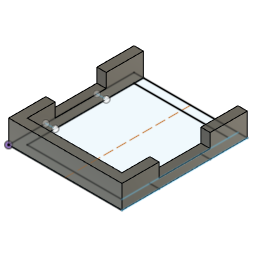
Final Project (Autodesk Fusion 360 design; units mm, degrees)
Autodesk Fusion 360 part; units mm, degrees
sketch "Sketch1" plane through (0, 0, 0) normal (0, 0, 1) x (1, 0, 0)
  line L0 (0, 0) -> (70, 0)
  line L1 (70, 0) -> (70, 120)
  line L2 (70, 120) -> (0, 120)
  line L3 (0, 120) -> (0, 0)
  dimension "d1" = 70
  dimension "d2" = 120
  constraint horizontal L0
  constraint vertical L1
  constraint horizontal L2
  constraint vertical L3
  constraint coincident L0.start L3.end
  measures "d1" distance of L0.start L0.end
  measures "d2" distance of L0.start L2.end
extrude "Extrude1" add sketch "Sketch1" along normal blind 25 makes body 1
sketch "Sketch2" plane through (0, 0, 25) normal (0, 0, 1) x (-1, 0, 0)
  line L0 (0, -120) -> (0, 0)
  line L1 (0, 0) -> (-70, 0)
  line L2 (-70, 0) -> (-70, -120)
  line L3 (-70, -120) -> (0, -120)
  line L4 (-5, -115) -> (-65, -115)
  line L5 (-65, -115) -> (-65, -5)
  line L6 (-65, -5) -> (-5, -5)
  line L7 (-5, -5) -> (-5, -115)
  dimension "d5" = 60
  dimension "d6" = 110
  dimension "d7" = 5
  dimension "d8" = 5
  constraint horizontal L4
  constraint vertical L5
  constraint horizontal L6
  constraint vertical L7
  measures "d5" distance of L4.start L4.end
  measures "d6" distance of L4.start L6.end
  measures "d7" distance of L2 L5
  measures "d8" distance of L1 L6
extrude "Extrude2" cut sketch "Sketch2" against normal blind 5 contours L4 L5 L6 L7 bodies 1
shell "Shell1" thickness 3 removed faces 1 at (23.3333, 80, 0) on bodies 1
sketch "Plate Sketch" plane through (0, 0, 17) normal (0, 0, -1) x (1, 0, 0)
  line L0 (3, -3) -> (3, -117)
  line L1 (3, -117) -> (67, -117)
  line L2 (67, -117) -> (67, -3)
  line L3 (67, -3) -> (3, -3)
  line L4 (8.9, -24) -> (23.1, -24)
  line L5 (23.1, -24) -> (23.1, -9.8)
  line L6 (23.1, -9.8) -> (8.9, -9.8)
  line L7 (8.9, -9.8) -> (8.9, -24)
  line L8 (3, -81) -> (67, -81) construction
  line L9 (61.1, -117) -> (61.1, -3) construction
  line L10 (27.9, -9.8) -> (27.9, -24)
  line L11 (27.9, -24) -> (42.1, -24)
  line L12 (42.1, -24) -> (42.1, -9.8)
  line L13 (42.1, -9.8) -> (27.9, -9.8)
  line L14 (46.9, -9.8) -> (46.9, -24)
  line L15 (46.9, -24) -> (61.1, -24)
  line L16 (61.1, -24) -> (61.1, -9.8)
  line L17 (61.1, -9.8) -> (46.9, -9.8)
  line L18 (8.9, -28.8) -> (8.9, -43)
  line L19 (8.9, -43) -> (23.1, -43)
  line L20 (23.1, -43) -> (23.1, -28.8)
  line L21 (23.1, -28.8) -> (8.9, -28.8)
  line L22 (27.9, -28.8) -> (27.9, -43)
  line L23 (27.9, -43) -> (42.1, -43)
  line L24 (42.1, -43) -> (42.1, -28.8)
  line L25 (42.1, -28.8) -> (27.9, -28.8)
  line L26 (46.9, -28.8) -> (46.9, -43)
  line L27 (46.9, -43) -> (61.1, -43)
  line L28 (61.1, -43) -> (61.1, -28.8)
  line L29 (61.1, -28.8) -> (46.9, -28.8)
  line L30 (8.9, -47.8) -> (8.9, -62)
  line L31 (8.9, -62) -> (23.1, -62)
  line L32 (23.1, -62) -> (23.1, -47.8)
  line L33 (23.1, -47.8) -> (8.9, -47.8)
  line L34 (27.9, -47.8) -> (27.9, -62)
  line L35 (27.9, -62) -> (42.1, -62)
  line L36 (42.1, -62) -> (42.1, -47.8)
  line L37 (42.1, -47.8) -> (27.9, -47.8)
  line L38 (46.9, -47.8) -> (46.9, -62)
  line L39 (46.9, -62) -> (61.1, -62)
  line L40 (61.1, -62) -> (61.1, -47.8)
  line L41 (61.1, -47.8) -> (46.9, -47.8)
  line L42 (8.9, -66.8) -> (8.9, -81)
  line L43 (8.9, -81) -> (23.1, -81)
  line L44 (23.1, -81) -> (23.1, -66.8)
  line L45 (23.1, -66.8) -> (8.9, -66.8)
  line L46 (27.9, -66.8) -> (27.9, -81)
  line L47 (27.9, -81) -> (42.1, -81)
  line L48 (42.1, -81) -> (42.1, -66.8)
  line L49 (42.1, -66.8) -> (27.9, -66.8)
  line L50 (46.9, -66.8) -> (46.9, -81)
  line L51 (46.9, -81) -> (61.1, -81)
  line L52 (61.1, -81) -> (61.1, -66.8)
  line L53 (61.1, -66.8) -> (46.9, -66.8)
  line L54 (46.9, -106.3141) -> (61.1, -106.3141)
  line L55 (61.1, -106.3141) -> (61.1, -92.1141)
  line L56 (61.1, -92.1141) -> (46.9, -92.1141)
  line L57 (46.9, -92.1141) -> (46.9, -106.3141)
  line L58 (46.9, -106.3141) -> (61.1, -92.1141) construction
  line L59 (61.1, -106.3141) -> (46.9, -92.1141) construction
  circle A0 centre (54, -99.2141) radius 3.5
  line L60 (9.0541, -114.2194) -> (34.0541, -114.2194) construction
  line L61 (34.0541, -114.2194) -> (34.0541, -87.2194) construction
  line L62 (34.0541, -87.2194) -> (9.0541, -87.2194) construction
  line L63 (9.0541, -87.2194) -> (9.0541, -114.2194) construction
  dimension "d18" = 14.2
  dimension "d19" = 14.2
  dimension "d20" = 6.8
  dimension "d21" = 5.9
  dimension "d23" = 5.9
  dimension "d24" = 71.2
  dimension "d27" = 38
  dimension "d28" = -57
  dimension "d29" = 14.2
  dimension "d30" = 14.2
  dimension "d32" = 5.9
  dimension "d33" = 7
  dimension "d34" = 25
  dimension "d35" = 27
  constraint horizontal L4
  constraint vertical L5
  constraint horizontal L6
  constraint vertical L7
  constraint coincident L0 L8.start
  constraint coincident L2 L8.end
  constraint perpendicular L2 L8
  constraint coincident L1 L9.start
  constraint coincident L3 L9.end
  constraint perpendicular L3 L9
  constraint horizontal L54
  constraint vertical L55
  constraint horizontal L56
  constraint vertical L57
  constraint midpoint L59 A0.centre
  constraint horizontal L60
  constraint vertical L61
  constraint horizontal L62
  constraint vertical L63
  measures "d18" distance of L4.start L4.end
  measures "d19" distance of L4.start L6.end
  measures "d20" distance of L3 L6
  measures "d21" distance of L0 L7
  measures "d23" distance of L2 L9
  measures "d24" distance of L6 L8
  measures "d29" distance of L54.start L54.end
  measures "d30" distance of L54.start L56.end
  measures "d32" distance of L2 L55
  measures "d33" diameter of A0
  measures "d34" distance of L60.start L60.end
  measures "d35" distance of L60.start L62.end
extrude "Extrude3" cut sketch "Plate Sketch" against normal blind 3 contours L0 L1 L2 L3 | L4 L5 L6 L7 | L10 L11 L12 L13 | L14 L15 L16 L17 | L18 L19 L20 L21 | L22 L23 L24 L25 | L26 L27 L28 L29 | L30 L31 L32 L33 | L34 L35 L36 L37 | L38 L39 L40 L41 | L42 L43 L44 L45 | L46 L47 L48 L49 | L50 L51 L52 L53 | L54 L55 L56 L57 | A0 bodies 1
extrude "Extrude4" add sketch "Plate Sketch" against normal blind 3 separate body contours L0 L1 L2 L3 | L54 L55 L56 L57 makes body 2
extrude "Extrude9" add 1 faces at (23.3333, 0, 8.3333) along direction (0, -1, 0) blind 5 on bodies 1 bodies 1
extrude "Extrude10" add 1 faces at (46.6667, 120, 8.3333) along direction (0, 1, 0) blind 5 on bodies 1 bodies 1
extrude "Extrude11" add 1 faces at (24.3333, 122.3333, 0) along direction (0, 0, -1) blind 2 separate body on bodies 1 makes body 3
extrude "Extrude12" add 1 faces at (24.3333, 117, -0.6667) along direction (0, -1, 0) blind 114 on bodies 3 bodies 3
sketch "Base Sketch" plane through (0, 0, 0) normal (0, 0, 1) x (-1, 0, 0)
  line L0 (0, -125) -> (0, 5)
  line L1 (0, 5) -> (-70, 5)
  line L2 (-70, 5) -> (-70, -125)
  line L3 (-70, -125) -> (0, -125)
  line L4 (-61.1, -66.8) -> (-46.9, -66.8)
  line L5 (-46.9, -66.8) -> (-46.9, -81)
  line L6 (-46.9, -81) -> (-61.1, -81)
  line L7 (-61.1, -81) -> (-61.1, -66.8)
  circle A0 centre (-54, -99.2141) radius 3.5
  line L8 (-23.1, -66.8) -> (-8.9, -66.8)
  line L9 (-8.9, -66.8) -> (-8.9, -81)
  line L10 (-8.9, -81) -> (-23.1, -81)
  line L11 (-23.1, -81) -> (-23.1, -66.8)
  line L12 (-23.1, -47.8) -> (-8.9, -47.8)
  line L13 (-8.9, -47.8) -> (-8.9, -62)
  line L14 (-8.9, -62) -> (-23.1, -62)
  line L15 (-23.1, -62) -> (-23.1, -47.8)
  line L16 (-42.1, -28.8) -> (-27.9, -28.8)
  line L17 (-27.9, -28.8) -> (-27.9, -43)
  line L18 (-27.9, -43) -> (-42.1, -43)
  line L19 (-42.1, -43) -> (-42.1, -28.8)
  line L20 (-42.1, -9.8) -> (-27.9, -9.8)
  line L21 (-27.9, -9.8) -> (-27.9, -24)
  line L22 (-27.9, -24) -> (-42.1, -24)
  line L23 (-42.1, -24) -> (-42.1, -9.8)
  line L24 (-23.1, -28.8) -> (-8.9, -28.8)
  line L25 (-8.9, -28.8) -> (-8.9, -43)
  line L26 (-8.9, -43) -> (-23.1, -43)
  line L27 (-23.1, -43) -> (-23.1, -28.8)
  line L28 (-61.1, -9.8) -> (-46.9, -9.8)
  line L29 (-46.9, -9.8) -> (-46.9, -24)
  line L30 (-46.9, -24) -> (-61.1, -24)
  line L31 (-61.1, -24) -> (-61.1, -9.8)
  line L32 (-8.9, -9.8) -> (-8.9, -24)
  line L33 (-8.9, -24) -> (-23.1, -24)
  line L34 (-23.1, -24) -> (-23.1, -9.8)
  line L35 (-23.1, -9.8) -> (-8.9, -9.8)
  line L36 (-61.1, -28.8) -> (-46.9, -28.8)
  line L37 (-46.9, -28.8) -> (-46.9, -43)
  line L38 (-46.9, -43) -> (-61.1, -43)
  line L39 (-61.1, -43) -> (-61.1, -28.8)
  line L40 (-61.1, -47.8) -> (-46.9, -47.8)
  line L41 (-46.9, -47.8) -> (-46.9, -62)
  line L42 (-46.9, -62) -> (-61.1, -62)
  line L43 (-61.1, -62) -> (-61.1, -47.8)
  line L44 (-3, -3) -> (-67, -3)
  line L45 (-67, -3) -> (-67, -117)
  line L46 (-67, -117) -> (-3, -117)
  line L47 (-3, -117) -> (-3, -3)
  line L48 (-61.1, -3) -> (-61.1, -117)
  line L49 (-8.9, -3) -> (-8.9, -117)
  line L50 (-8.9, -3) -> (-8.9, 5) construction
  line L51 (-61.1, -3) -> (-61.1, 5) construction
  line L52 (-8.9, -117) -> (-8.9, -125) construction
  line L53 (-61.1, -117) -> (-61.1, -125) construction
  circle A1 centre (-61.1, 1) radius 2.75
  circle A2 centre (-8.9, 1) radius 2.75
  circle A3 centre (-61.1, -121) radius 2.75
  circle A4 centre (-8.9, -121) radius 2.75
  line L54 (-35, -117) -> (-35, -82.6312) construction
  line L55 (-41, -117) -> (-29, -117)
  line L56 (-29, -117) -> (-29, -72)
  line L57 (-29, -72) -> (-41, -72)
  line L58 (-41, -72) -> (-41, -117)
  line L59 (-35, -117) -> (-35, -110) construction
  dimension "d90" = 5.5
  dimension "d91" = 5.5
  dimension "d92" = 5.5
  dimension "d93" = 5.5
  dimension "d107" = 12
  dimension "d108" = 45
  constraint coincident L44 L48.start
  constraint coincident L46 L48.end
  constraint perpendicular L46 L48
  constraint coincident L44 L49.start
  constraint coincident L46 L49.end
  constraint perpendicular L46 L49
  constraint coincident L1 L50.end
  constraint perpendicular L1 L50
  constraint coincident L1 L51.end
  constraint perpendicular L1 L51
  constraint coincident L3 L52.end
  constraint perpendicular L3 L52
  constraint coincident L3 L53.end
  constraint perpendicular L3 L53
  constraint midpoint L51 A1.centre
  constraint midpoint L50 A2.centre
  constraint midpoint L53 A3.centre
  constraint midpoint L52 A4.centre
  constraint midpoint L46 L54.start
  constraint perpendicular L46 L54
  constraint horizontal L55
  constraint vertical L56
  constraint horizontal L57
  constraint vertical L58
  constraint coincident L46 L55.start
  constraint midpoint L55 L54.start
  constraint perpendicular L46 L59
  constraint collinear L54 L59
  measures "d90" diameter of A1
  measures "d91" diameter of A2
  measures "d92" diameter of A3
  measures "d93" diameter of A4
  measures "d107" distance of L55.start L55.end
  measures "d108" distance of L55.start L57.end
extrude "Extrude23" add sketch "Base Sketch" along normal blind 3 contours L46 L55 L56 L57 L58 bodies 3
extrude "Extrude13" add sketch "Base Sketch" along normal blind 17 contours L7 L31 L39 L43 L44 L45 L46 L48 bodies 3
extrude "Extrude14" add sketch "Base Sketch" along normal blind 17 contours L9 L13 L25 L32 L44 L46 L47 L49 bodies 3
extrude "Extrude7" add 1 faces at (45.6667, 117, 6.6667) along direction (0, -1, 0) blind 5 on bodies 1 bodies 1
extrude "Extrude8" add 1 faces at (24.3333, 3, 6.6667) along direction (0, 1, 0) blind 5 on bodies 1 bodies 1
fillet "Fillet2" radius 5 4 edges at (70, -5, 12.5) (0, -5, 12.5) (0, 125, 12.5) (70, 125, 12.5) on bodies 1
fillet "Fillet3" radius 1 8 edges at (0, 60, 25) (1.4645, 123.5355, 25) (35, 125, 25) (68.5355, 123.5355, 25) (70, 60, 25) (68.5355, -3.5355, 25) (35, -5, 25) (1.4645, -3.5355, 25) on bodies 1
fillet "Fillet4" radius 5 4 edges at (0, 125, -1) (70, 125, -1) (70, -5, -1) (0, -5, -1) on bodies 3
extrude "Extrude15" cut 1 faces at (25, 8, 6.6667) along direction (0, -1, 0) blind 3 on bodies 1 bodies 1
extrude "Extrude16" cut 1 faces at (45, 112, 6.6667) along direction (0, 1, 0) blind 3 on bodies 1 bodies 1
combine "Combine1" operation cut target body 1 tool bodies 2 keep tools
extrude "Extrude17" cut 1 faces at (45.6667, 115, 5.6667) along direction (0, 1, 0) blind 2 on bodies 1 bodies 1
extrude "Extrude18" cut 1 faces at (24.3333, 5, 5.6667) along direction (0, -1, 0) blind 2 on bodies 1 bodies 1
sketch "Plate Sketch Modified" plane through (0, 0, 20) normal (0, 0, 1) x (-1, 0, 0)
  line L0 (-23.1, -28.8) -> (-8.9, -28.8)
  line L1 (-8.9, -28.8) -> (-8.9, -43)
  line L2 (-8.9, -43) -> (-23.1, -43)
  line L3 (-23.1, -43) -> (-23.1, -28.8)
  line L4 (-61.1, -28.8) -> (-46.9, -28.8)
  line L5 (-46.9, -28.8) -> (-46.9, -43)
  line L6 (-46.9, -43) -> (-61.1, -43)
  line L7 (-61.1, -43) -> (-61.1, -28.8)
  circle A0 centre (-54, -99.2141) radius 3.5
  line L8 (-8.9, -9.8) -> (-8.9, -24)
  line L9 (-8.9, -24) -> (-23.1, -24)
  line L10 (-23.1, -24) -> (-23.1, -9.8)
  line L11 (-23.1, -9.8) -> (-8.9, -9.8)
  line L12 (-42.1, -47.8) -> (-27.9, -47.8)
  line L13 (-27.9, -47.8) -> (-27.9, -62)
  line L14 (-27.9, -62) -> (-42.1, -62)
  line L15 (-42.1, -62) -> (-42.1, -47.8)
  line L16 (-61.1, -47.8) -> (-46.9, -47.8)
  line L17 (-46.9, -47.8) -> (-46.9, -62)
  line L18 (-46.9, -62) -> (-61.1, -62)
  line L19 (-61.1, -62) -> (-61.1, -47.8)
  line L20 (-42.1, -66.8) -> (-27.9, -66.8)
  line L21 (-27.9, -66.8) -> (-27.9, -81)
  line L22 (-27.9, -81) -> (-42.1, -81)
  line L23 (-42.1, -81) -> (-42.1, -66.8)
  line L24 (-61.1, -66.8) -> (-46.9, -66.8)
  line L25 (-46.9, -66.8) -> (-46.9, -81)
  line L26 (-46.9, -81) -> (-61.1, -81)
  line L27 (-61.1, -81) -> (-61.1, -66.8)
  line L28 (-23.1, -47.8) -> (-8.9, -47.8)
  line L29 (-8.9, -47.8) -> (-8.9, -62)
  line L30 (-8.9, -62) -> (-23.1, -62)
  line L31 (-23.1, -62) -> (-23.1, -47.8)
  line L32 (-42.1, -9.8) -> (-27.9, -9.8)
  line L33 (-27.9, -9.8) -> (-27.9, -24)
  line L34 (-27.9, -24) -> (-42.1, -24)
  line L35 (-42.1, -24) -> (-42.1, -9.8)
  line L36 (-23.1, -66.8) -> (-8.9, -66.8)
  line L37 (-8.9, -66.8) -> (-8.9, -81)
  line L38 (-8.9, -81) -> (-23.1, -81)
  line L39 (-23.1, -81) -> (-23.1, -66.8)
  line L40 (-61.1, -9.8) -> (-46.9, -9.8)
  line L41 (-46.9, -9.8) -> (-46.9, -24)
  line L42 (-46.9, -24) -> (-61.1, -24)
  line L43 (-61.1, -24) -> (-61.1, -9.8)
  line L44 (-42.1, -28.8) -> (-27.9, -28.8)
  line L45 (-27.9, -28.8) -> (-27.9, -43)
  line L46 (-27.9, -43) -> (-42.1, -43)
  line L47 (-42.1, -43) -> (-42.1, -28.8)
  line L48 (-3, -3) -> (-67, -3)
  line L49 (-67, -3) -> (-67, -117)
  line L50 (-67, -117) -> (-3, -117)
  line L51 (-3, -117) -> (-3, -3)
  line L52 (-9, -66.9) -> (-9, -80.9)
  line L53 (-9, -80.9) -> (-23, -80.9)
  line L54 (-23, -80.9) -> (-23, -66.9)
  line L55 (-23, -66.9) -> (-9, -66.9)
  line L56 (-42, -66.9) -> (-28, -66.9)
  line L57 (-28, -66.9) -> (-28, -80.9)
  line L58 (-28, -80.9) -> (-42, -80.9)
  line L59 (-42, -80.9) -> (-42, -66.9)
  line L60 (-61, -66.9) -> (-47, -66.9)
  line L61 (-47, -66.9) -> (-47, -80.9)
  line L62 (-47, -80.9) -> (-61, -80.9)
  line L63 (-61, -80.9) -> (-61, -66.9)
  line L64 (-23, -47.9) -> (-9, -47.9)
  line L65 (-9, -47.9) -> (-9, -61.9)
  line L66 (-9, -61.9) -> (-23, -61.9)
  line L67 (-23, -61.9) -> (-23, -47.9)
  line L68 (-42, -47.9) -> (-28, -47.9)
  line L69 (-28, -47.9) -> (-28, -61.9)
  line L70 (-28, -61.9) -> (-42, -61.9)
  line L71 (-42, -61.9) -> (-42, -47.9)
  line L72 (-61, -47.9) -> (-47, -47.9)
  line L73 (-47, -47.9) -> (-47, -61.9)
  line L74 (-47, -61.9) -> (-61, -61.9)
  line L75 (-61, -61.9) -> (-61, -47.9)
  line L76 (-23, -28.9) -> (-9, -28.9)
  line L77 (-9, -28.9) -> (-9, -42.9)
  line L78 (-9, -42.9) -> (-23, -42.9)
  line L79 (-23, -42.9) -> (-23, -28.9)
  line L80 (-42, -28.9) -> (-28, -28.9)
  line L81 (-28, -28.9) -> (-28, -42.9)
  line L82 (-28, -42.9) -> (-42, -42.9)
  line L83 (-42, -42.9) -> (-42, -28.9)
  line L84 (-61, -28.9) -> (-47, -28.9)
  line L85 (-47, -28.9) -> (-47, -42.9)
  line L86 (-47, -42.9) -> (-61, -42.9)
  line L87 (-61, -42.9) -> (-61, -28.9)
  line L88 (-23, -9.9) -> (-9, -9.9)
  line L89 (-9, -9.9) -> (-9, -23.9)
  line L90 (-9, -23.9) -> (-23, -23.9)
  line L91 (-23, -23.9) -> (-23, -9.9)
  line L92 (-42, -9.9) -> (-28, -9.9)
  line L93 (-28, -9.9) -> (-28, -23.9)
  line L94 (-28, -23.9) -> (-42, -23.9)
  line L95 (-42, -23.9) -> (-42, -9.9)
  line L96 (-61, -9.9) -> (-47, -9.9)
  line L97 (-47, -9.9) -> (-47, -23.9)
  line L98 (-47, -23.9) -> (-61, -23.9)
  line L99 (-61, -23.9) -> (-61, -9.9)
  circle A1 centre (-54, -99.2141) radius 3.5
  line L100 (-12.5, -112.4) -> (-37.5, -112.4) construction
  line L101 (-37.5, -112.4) -> (-37.5, -85.4) construction
  line L102 (-37.5, -85.4) -> (-12.5, -85.4) construction
  line L103 (-12.5, -85.4) -> (-12.5, -112.4) construction
  line L104 (-20, -112.4) -> (-30, -112.4)
  line L105 (-30, -112.4) -> (-30, -109.4)
  line L106 (-30, -109.4) -> (-20, -109.4)
  line L107 (-20, -109.4) -> (-20, -112.4)
  dimension "d70" = 0.1
  dimension "d71" = 0.1
  dimension "d72" = 0.1
  dimension "d73" = 0.1
  dimension "d74" = 0.1
  dimension "d75" = 0.1
  dimension "d76" = 0.1
  dimension "d77" = 0.1
  dimension "d78" = 0.1
  dimension "d79" = 0.1
  dimension "d80" = 0.1
  dimension "d81" = 0.1
  dimension "d82" = 25
  dimension "d83" = 27
  dimension "d84" = 4.6
  dimension "d85" = 9.5
  dimension "d86" = 10
  dimension "d87" = 3
  dimension "d88" = 7.5
  constraint horizontal L100
  constraint vertical L101
  constraint horizontal L102
  constraint vertical L103
  constraint horizontal L104
  constraint vertical L105
  constraint horizontal L106
  constraint vertical L107
  constraint coincident L100 L104.start
  measures "d82" distance of L100.start L100.end
  measures "d83" distance of L100.start L102.end
  measures "d84" distance of L50 L100
  measures "d85" distance of L51 L103
  measures "d86" distance of L104.start L104.end
  measures "d87" distance of L104.start L106.end
  measures "d88" distance of L101 L105
extrude "Extrude19" add 1 faces at (46.6667, 40, -2) along direction (0, 0, -1) blind 1 on bodies 3 bodies 3
sketch "Base Sketch 2" plane through (0, 0, -3) normal (0, 0, -1) x (1, 0, 0)
  arc A0 (5, 5) -> (0, 0) centre (5, 0) ccw
  line L0 (0, 0) -> (0, -120)
  arc A1 (0, -120) -> (5, -125) centre (5, -120) ccw
  line L1 (5, -125) -> (65, -125)
  arc A2 (65, -125) -> (70, -120) centre (65, -120) ccw
  line L2 (70, -120) -> (70, 0)
  arc A3 (70, 0) -> (65, 5) centre (65, 0) ccw
  line L3 (65, 5) -> (5, 5)
  circle A4 centre (61.1, -121) radius 2.75
  circle A5 centre (8.9, -121) radius 2.75
  circle A6 centre (8.9, 1) radius 2.75
  circle A7 centre (61.1, 1) radius 2.75
  circle A8 centre (61.1, 1) radius 1.5
  circle A9 centre (8.9, 1) radius 1.5
  circle A10 centre (61.1, -121) radius 1.5
  circle A11 centre (8.9, -121) radius 1.5
  dimension "d101" = 3
  dimension "d102" = 3
  dimension "d103" = 3
  dimension "d104" = 3
  constraint concentric A7 A8
  constraint concentric A6 A9
  constraint concentric A4 A10
  constraint concentric A5 A11
  measures "d101" diameter of A8
  measures "d102" diameter of A9
  measures "d103" diameter of A10
  measures "d104" diameter of A11
extrude "Extrude20" cut sketch "Base Sketch 2" against normal blind 2 contours A4 | A5 | A6 | A7 | A8 | A9 | A10 | A11 bodies 3
extrude "Extrude21" add sketch "Base Sketch" along normal blind 2 contours A1 | A2 | A3 | A4 bodies 3
extrude "Extrude22" cut sketch "Base Sketch 2" against normal blind 5 contours A8 | A9 | A10 | A11 bodies 3
sketch "Pi Pico" plane through (0, 0, 3) normal (0, 0, 1) x (-1, 0, 0)
  line L0 (-41, -72) -> (-41, -117)
  line L1 (-41, -117) -> (-29, -117)
  line L2 (-29, -117) -> (-29, -72)
  line L3 (-29, -72) -> (-41, -72)
  line L4 (-24.5, -117) -> (-45.5, -117)
  line L5 (-45.5, -117) -> (-45.5, -66)
  line L6 (-45.5, -66) -> (-24.5, -66)
  line L7 (-24.5, -66) -> (-24.5, -117)
  line L8 (-67, -117) -> (-3, -117)
  line L9 (-35, -117) -> (-35, -113) construction
  line L10 (-35, -117) -> (-35, -110)
  line L11 (-31, -118) -> (-39, -118)
  line L12 (-39, -118) -> (-39, -117)
  line L13 (-39, -117) -> (-31, -117)
  line L14 (-31, -117) -> (-31, -118)
  line L15 (-35, -118) -> (-35, -117) construction
  dimension "d111" = 21
  dimension "d112" = 51
  dimension "d115" = 8
  dimension "d116" = 1
  constraint horizontal L4
  constraint vertical L5
  constraint horizontal L6
  constraint vertical L7
  constraint collinear L4 L8
  constraint midpoint L4 L9.start
  constraint perpendicular L4 L9
  constraint collinear L9 L10
  constraint horizontal L11
  constraint vertical L12
  constraint horizontal L13
  constraint vertical L14
  constraint midpoint L11 L15.start
  constraint midpoint L13 L9.start
  constraint collinear L10 L15
  constraint collinear L4 L13
  measures "d111" distance of L4.start L4.end
  measures "d112" distance of L4.start L6.end
  measures "d115" distance of L11.start L11.end
  measures "d116" distance of L11.start L13.end
extrude "Extrude24" add sketch "Pi Pico" along normal blind 1 separate body contours L0 L1 L2 L3 L4 L8 L13 | L0 L2 L3 L4 L5 L6 L7 L8 makes body 4
extrude "Extrude25" add sketch "Pi Pico" along normal blind 2 contours L1 L4 L8 L11 L12 L13 L14 bodies 4
extrude "Extrude26" cut sketch "Pi Pico" along normal blind 1 contours L1 L4 L8 L11 L12 L13 L14 bodies 4
extrude "Extrude27" add 1 faces at (36.3333, 117, 4.6667) along direction (0, -1, 0) blind 4.3 on bodies 4 bodies 4
fillet "Fillet5" radius 2 4 edges at (65, 115, 22.5) (5, 115, 22.5) (5, 5, 22.5) (65, 5, 22.5) on bodies 1
combine "Combine2" operation cut target body 1 tool bodies 3 keep tools
extrude "Extrude28" cut 4 faces at (61.0626, 122.0619, 0) (8.5335, 120.3652, 0) (9.3778, -1.5328, 0) (60.4395, -1.3621, 0) along direction (0, 0, 1) blind 8 on bodies 1 bodies 1
extrude "Extrude29" add 1 faces at (33, 72, 1) along direction (0, -1, 0) blind 6 on bodies 3 bodies 3
extrude "Extrude30" add 1 faces at (33, 66, 1) along direction (0, -1, 0) blind 1 on bodies 3 bodies 3
sketch "Sketch12" plane through (0, 0, 3) normal (0, 0, 1) x (-1, 0, 0)
  line L0 (-41, -65) -> (-41, -117)
  line L1 (-41, -117) -> (-29, -117)
  line L2 (-29, -117) -> (-29, -65)
  line L3 (-29, -65) -> (-41, -65)
  line L4 (-41, -66) -> (-29, -66)
  dimension "d131" = 1
  constraint coincident L0 L4.start
  constraint coincident L2 L4.end
  constraint perpendicular L2 L4
  measures "d131" distance of L3 L4
extrude "Extrude31" add sketch "Sketch12" along normal blind 2 contours L0 L2 L3 L4 bodies 3
sketch "Sketch13" plane through (0, 66, 0) normal (0, 1, 0) x (-1, 0, 0)
  line L0 (-41, 3) -> (-29, 3)
  line L1 (-29, 3) -> (-29, 5)
  line L2 (-29, 5) -> (-41, 5)
  line L3 (-41, 5) -> (-41, 3)
  line L4 (-41, 4) -> (-29, 4)
  constraint midpoint L3 L4.start
  constraint midpoint L1 L4.end
extrude "Extrude32" add sketch "Sketch13" along normal blind 1 contours L1 L2 L3 L4 bodies 3
extrude "Extrude33" add 1 faces at (36.3333, 116.2333, 5) along direction (0, 0, 1) blind 2 on bodies 4 bodies 4
extrude "Extrude34" add 1 faces at (33.6667, 118, 5) along direction (0, 1, 0) blind 65 on bodies 4 bodies 4
extrude "Extrude35" cut 1 faces at (33.6667, 183, 5) along direction (0, -1, 0) blind 57 on bodies 4 bodies 4
extrude "Extrude36" cut 1 faces at (33.6667, 126, 5) along direction (0, -1, 0) blind 1 on bodies 4 bodies 4
sketch "Sketch14" plane through (0, 125, 0) normal (0, 1, 0) x (-1, 0, 0)
  line L0 (-5, 24) -> (-65, 24)
  line L1 (-65, 24) -> (-65, 0)
  line L2 (-65, 0) -> (-5, 0)
  line L3 (-5, 0) -> (-5, 24)
  line L4 (-31, 7) -> (-31, 4)
  line L5 (-39, 7) -> (-31, 7)
  line L6 (-39, 4) -> (-39, 7)
  line L7 (-31, 4) -> (-39, 4)
  line L8 (-31, 2) -> (-39, 2)
  line L9 (-41, 4) -> (-41, 7)
  line L10 (-39, 9) -> (-31, 9)
  line L11 (-29, 7) -> (-29, 4)
  arc A0 (-29, 7) -> (-31, 9) centre (-31, 7) ccw
  arc A1 (-41, 4) -> (-39, 2) centre (-39, 4) ccw
  arc A2 (-39, 9) -> (-41, 7) centre (-39, 7) ccw
  arc A3 (-31, 2) -> (-29, 4) centre (-31, 4) ccw
  line L12 (-31.5, 3.5) -> (-38.5, 3.5)
  line L13 (-39.5, 4.5) -> (-39.5, 6.5)
  line L14 (-38.5, 7.5) -> (-31.5, 7.5)
  line L15 (-30.5, 6.5) -> (-30.5, 4.5)
  arc A4 (-38.5, 7.5) -> (-39.5, 6.5) centre (-38.5, 6.5) ccw
  arc A5 (-30.5, 6.5) -> (-31.5, 7.5) centre (-31.5, 6.5) ccw
  arc A6 (-31.5, 3.5) -> (-30.5, 4.5) centre (-31.5, 4.5) ccw
  arc A7 (-39.5, 4.5) -> (-38.5, 3.5) centre (-38.5, 4.5) ccw
  dimension "d145" = 2
  dimension "d146" = 2
  dimension "d149" = 2
  dimension "d151" = 1
  dimension "d152" = 1
  dimension "d153" = 1
  dimension "d154" = 1
  constraint parallel L7 L8
  constraint parallel L6 L9
  constraint parallel L5 L10
  constraint parallel L4 L11
  constraint tangent L10 A0
  constraint tangent L11 A0
  constraint tangent L9 A1
  constraint tangent L8 A1
  constraint tangent L10 A2
  constraint tangent L9 A2
  constraint equal A1 A2
  constraint tangent L8 A3
  constraint tangent L11 A3
  constraint parallel L7 L12
  constraint parallel L6 L13
  constraint parallel L5 L14
  constraint parallel L4 L15
  constraint tangent L14 A4
  constraint tangent L13 A4
  constraint tangent L14 A5
  constraint tangent L15 A5
  constraint tangent L15 A6
  constraint tangent L12 A6
  constraint tangent L13 A7
  constraint tangent L12 A7
  measures "d145" radius of A0
  measures "d146" radius of A1
  measures "d149" radius of A3
  measures "d151" radius of A4
  measures "d152" radius of A5
  measures "d153" radius of A6
  measures "d154" radius of A7
extrude "Extrude37" cut sketch "Sketch14" against normal blind 6 contours L4 L5 L6 L7 bodies 4
extrude "Extrude38" cut sketch "Sketch14" against normal blind 12 contours L4 L5 L6 L7 | L12 L13 L14 L15 A4 A5 A6 A7 bodies 1
extrude "Extrude39" cut sketch "Sketch14" against normal blind 6 contours L8 L9 L10 L11 A0 A1 A2 A3 bodies 1
extrude "Extrude40" add sketch "Plate Sketch Modified" against normal blind 3 separate body contours L48 L49 L50 L51 makes body 5
extrude "Extrude41" cut 1 faces at (67, 41, 6.6667) along direction (1, 0, 0) blind 0.5 on bodies 1 bodies 1
extrude "Extrude42" cut 1 faces at (58.1633, 117, 8.8808) along direction (0, 1, 0) blind 0.5 on bodies 1 bodies 1
extrude "Extrude43" cut 1 faces at (3, 41.1667, 13.3333) along direction (-1, 0, 0) blind 0.5 on bodies 1 bodies 1
extrude "Extrude44" cut 1 faces at (45.8333, 3, 13.3333) along direction (0, -1, 0) blind 0.5 on bodies 1 bodies 1
extrude "Extrude45" cut 1 faces at (66.6667, 77.6667, 20) along direction (0, 0, 1) blind 0.5 on bodies 1 bodies 1
extrude "Extrude46" add 2 faces at (6.9333, 41, 17) (65.0333, 79, 17) along direction (0, 0, 1) blind 0.3 on bodies 3 bodies 3
extrude "Extrude47" cut 1 faces at (33, 65.6667, 5) along direction (0, 0, -1) blind 2 on bodies 3 bodies 3
extrude "Extrude48" add 1 faces at (33, 65, 1) along direction (0, -1, 0) blind 2 on bodies 3 bodies 3
sketch "Sketch15" plane through (0, 0, 3) normal (0, 0, 1) x (-1, 0, 0)
  line L0 (-41, -63) -> (-41, -117)
  line L1 (-41, -117) -> (-29, -117)
  line L2 (-29, -117) -> (-29, -63)
  line L3 (-29, -63) -> (-41, -63)
  line L4 (-41, -65) -> (-29, -65)
  dimension "d177" = 2
  constraint coincident L0 L4.start
  constraint coincident L2 L4.end
  constraint perpendicular L0 L4
  measures "d177" distance of L3 L4
extrude "Extrude49" add sketch "Sketch15" along normal blind 3.5 contours L0 L2 L3 L4 bodies 3
sketch "Sketch16" plane through (0, 65, 0) normal (0, 1, 0) x (-1, 0, 0)
  line L0 (-41, 3) -> (-29, 3)
  line L1 (-29, 3) -> (-29, 6.5)
  line L2 (-29, 6.5) -> (-41, 6.5)
  line L3 (-41, 6.5) -> (-41, 3)
  line L4 (-41, 4.9983) -> (-29, 4.9983)
  constraint coincident L3 L4.start
  constraint coincident L1 L4.end
  constraint perpendicular L1 L4
extrude "Extrude50" add sketch "Sketch16" along normal blind 2 contours L1 L2 L3 L4 bodies 3
sketch "Sketch19" plane through (0, 0, 0) normal (0, 0, 1) x (1, 0, 0)
  line L0 (0, 0) -> (24.396, 0)
  line L1 (24.396, 0) -> (24.396, 27)
  line L2 (24.396, 27) -> (0, 27)
  line L3 (0, 27) -> (0, 0)
  line L4 (2, 2) -> (22.396, 2)
  line L5 (22.396, 2) -> (22.396, 25)
  line L6 (22.396, 25) -> (2, 25)
  line L7 (2, 25) -> (2, 2)
  line L8 (2, 25) -> (2, 27)
  line L9 (22.396, 25) -> (22.396, 27)
  line L10 (22.396, 8) -> (24.396, 8)
  line L11 (22.396, 19) -> (24.396, 19)
  line L12 (12.198, 27) -> (12.198, 0) construction
  line L13 (2, 19) -> (0, 19)
  line L14 (2, 8) -> (0, 8)
  dimension "d186" = 27
  dimension "d187" = -2
  dimension "d190" = 8
  dimension "d191" = 8
  constraint horizontal L0
  constraint vertical L1
  constraint horizontal L2
  constraint vertical L3
  constraint coincident L0.start L3.end
  constraint coincident L2 L8.end
  constraint perpendicular L2 L8
  constraint coincident L2 L9.end
  constraint perpendicular L2 L9
  constraint coincident L5 L10.start
  constraint coincident L1 L10.end
  constraint perpendicular L1 L10
  constraint coincident L5 L11.start
  constraint coincident L1 L11.end
  constraint perpendicular L1 L11
  constraint midpoint L2 L12.start
  constraint midpoint L0 L12.end
  constraint symmetric L10.start L12 L14.start
  constraint symmetric L10.end L12 L14.end
  constraint symmetric L11.start L12 L13.start
  constraint symmetric L11.end L12 L13.end
  measures "d186" distance of L0.start L2.end
  measures "d190" distance of L2 L11
  measures "d191" distance of L0 L10
extrude "Extrude53" add sketch "Sketch19" along normal blind 5 separate body contours L0 L1 L3 L4 L5 L7 L10 L14 | L2 L3 L7 L8 L13 | L1 L2 L5 L9 L11 makes body 6 at (8.132, 0, 1.6667) makes body 7 at (2, 21.6667, 1.6667) makes body 8 at (22.396, 21.6667, 1.6667)
extrude "Extrude54" add sketch "Sketch19" along normal blind 2 contours L3 L7 L13 L14 | L1 L5 L10 L11 bodies 6 7 8
hidden bodies 1 2 3 4 5
equation "d88 = ( ( 25 - 10 ) / 2 ) * 1 mm"
equation "screwOuterHole = 5.5 mm"
equation "d90 = screwOuterHole"
equation "d91 = screwOuterHole"
equation "d92 = screwOuterHole"
equation "d93 = screwOuterHole"
equation "screwInnerHole = 3 mm"
equation "d101 = screwInnerHole"
equation "d102 = screwInnerHole"
equation "d103 = screwInnerHole"
equation "d104 = screwInnerHole"
equation "d108 = 51 mm - 6 mm"
named bodies: "Top", "Plate", "Base", "Pi Pico", "Plate V2", "DIsplay Mount"
